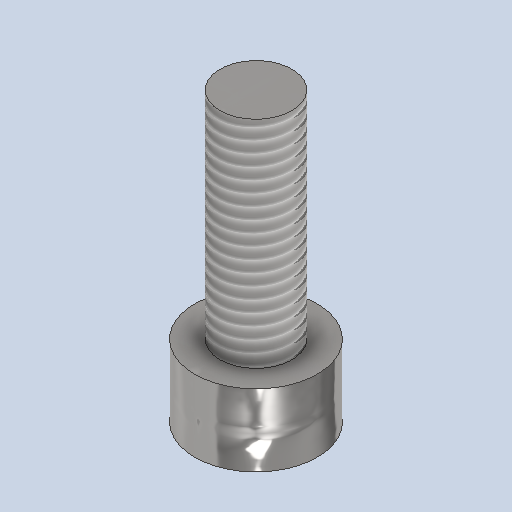
# Autodesk Inventor part: UC-0515
Saved by Autodesk Inventor 2024.2 (Build 282272000, 272)
## iProperties
Created: 2024-01-03
Part Number: UC-0515
Material: Stainless Steel AISI 304
Document SubType Name: Modeling
Designer: Masato Kubotera
Density: 8 g/cm^3
Appearance: Satin Hammered
Vendor: NISSAN SCREW
Mass: 4.34887 g
Surface Area: 5.17268 cm^2
Volume: 0.543608 cm^3
Catalog Web Link: https://wilco.jp/products/U/UC.html#page6
Author: Masato Kubotera
Autodesk Inventor part; units mm, degrees
ref_plane "YZ Plane" through (0, 0, 0) normal (1, 0, 0) x (0, 1, 0)
ref_plane "XZ Plane" through (0, 0, 0) normal (0, 1, 0) x (-1, 0, 0)
ref_plane "XY Plane" through (0, 0, 0) normal (0, 0, 1) x (1, 0, 0)
sketch "Sketch1" plane through (0, 0, 0) normal (0, 1, 0) x (-1, 0, 0)
  line L0 (0, 0) -> (-4.25, 0)
  line L1 (-4.25, 0) -> (-4.25, 5)
  line L2 (-4.25, 5) -> (-2.5, 5)
  line L3 (-2.5, 5) -> (-2.5, 20)
  line L4 (-2.5, 20) -> (0, 20)
  line L5 (0, 20) -> (0, 0)
  dimension "ScrewLength" = 15
  dimension "Diameter" = 8.5
  dimension "Metric" = 5
  dimension "HeadLength" = 5
  constraints: 12 end point, 3 horizontal, 3 vertical
  measures "ScrewLength" distance of L2.end L3.end
  measures "Diameter" diameter of L1 L5
  measures "Metric" diameter of L3 L5
  measures "HeadLength" distance of L0.end L1.end
revolve "Revolution1" add sketch "Sketch1" angle 360 about axis through (0, 0, 20) along (0, 0, -1)
thread "Thread1" size "M5x0.8" class "6g" standard "ANSI Metric M Profile" full length
sketch "Sketch2" plane through (0, 0, 0) normal (0, 0, -1) x (-1, 0, 0)
  line L0 (1.1547, 2) -> (2.3094, 0)
  line L1 (2.3094, 0) -> (1.1547, -2)
  line L2 (1.1547, -2) -> (-1.1547, -2)
  line L3 (-1.1547, -2) -> (-2.3094, 0)
  line L4 (-2.3094, 0) -> (-1.1547, 2)
  line L5 (-1.1547, 2) -> (1.1547, 2)
  point P0 (0, 0)
  point P1 (0, 0)
  dimension "WidthAcrossFlat" = 4
  constraints: 12 end point, 1 coincident, 1 horizontal, 13 other
  measures "WidthAcrossFlat" distance between parallel lines of L2 L5
extrude "Extrusion1" cut sketch "Sketch2" against normal blind 2.5
body "Solid1"
